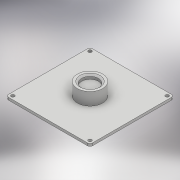
# Autodesk Inventor part: CAMERA
Saved by Autodesk Inventor 2017 (Build 210142000, 142)
## iProperties
Created: 2017-04-01
Part Number: CAMERA
Material: Generic
Document SubType Name: Modeling
Designer: Muchen
Density: 1 g/cm^3
Appearance: Default
Author: Muchen
Autodesk Inventor part; units mm, degrees
ref_plane "YZ Plane" through (0, 0, 0) normal (1, 0, 0) x (0, 1, 0)
ref_plane "XZ Plane" through (0, 0, 0) normal (0, 1, 0) x (-1, 0, 0)
ref_plane "XY Plane" through (0, 0, 0) normal (0, 0, 1) x (1, 0, 0)
sketch "Sketch1" plane through (0, 0, 0) normal (0, 0, 1) x (1, 0, 0)
  line L0 (3, 0) -> (97, 0)
  line L1 (100, 3) -> (100, 97)
  line L2 (97, 100) -> (3, 100)
  line L3 (0, 97) -> (0, 3)
  line L4 (4, 96) -> (96, 96) construction
  line L5 (96, 96) -> (96, 4) construction
  line L6 (96, 4) -> (4, 4) construction
  line L7 (4, 4) -> (4, 96) construction
  arc A0 (3, 100) -> (0, 97) centre (3, 97) ccw
  arc A1 (0, 3) -> (3, 0) centre (3, 3) ccw
  arc A2 (97, 0) -> (100, 3) centre (97, 3) ccw
  arc A3 (100, 97) -> (97, 100) centre (97, 97) ccw
  circle A4 centre (4, 96) radius 2
  circle A5 centre (4, 4) radius 2
  circle A6 centre (96, 4) radius 2
  circle A7 centre (96, 96) radius 2
  circle A8 centre (50, 50) radius 15
  circle A9 centre (50, 50) radius 10
  point P0 (0, 0)
  point P1 (100, 100)
  point P2 (100, 0)
  point P3 (0, 100)
  point P4 (50, 96)
  point P5 (4, 50)
  dimension "d0" = 100
  dimension "d1" = 100
  dimension "d2" = 4
  dimension "d3" = 3
  dimension "d4" = 4
  dimension "d5" = 20
  dimension "d6" = 30
  constraints: 16 end point, 10 centre point, 9 coincident, 8 point on circle, 8 point on line, 8 tangent, 6 equal radius, 4 parallel, 2 midpoint, 2 perpendicular, 1 horizontal, 1 horizontal alignment, 1 vertical alignment, 3 other
  measures "d0" distance of point (0, 100) point (100, 100)
  measures "d1" distance of point (100, 100) point (100, 0)
  measures "d2" distance between parallel lines of L2 L4
  measures "d3" radius of A0
  measures "d4" diameter of A6
  measures "d5" diameter of A9
  measures "d6" diameter of A8
extrude "Extrusion1" add sketch "Sketch1" against normal blind 3 contours A1 L3 A0 L2 A3 L1 A2 L0 | A8 | A9
extrude "Extrusion2" add sketch "Sketch1" along normal blind 15 contours A8
extrude "Extrusion3" add sketch "Sketch1" along normal blind 10 contours A9
chamfer "Chamfer1" distance 2 angle 45 1 edges at (40, 50, 15)
body "Solid1"
